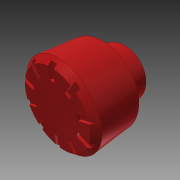
# Autodesk Inventor part: rotary_encoder_cnob
Saved by Autodesk Inventor 2014 (Build 180170000, 170)
## iProperties
Created: 2014-01-11
Part Number: rotary_encoder_cnob
Material: ABS Plastic
Document SubType Name: Modeling
Designer: buben
Density: 1.06 g/cm^3
Appearance: Light Red
Author: buben
Autodesk Inventor part; units mm, degrees
ref_plane "YZ Plane" through (0, 0, 0) normal (1, 0, 0) x (0, 1, 0)
ref_plane "XZ Plane" through (0, 0, 0) normal (0, 1, 0) x (-1, 0, 0)
ref_plane "XY Plane" through (0, 0, 0) normal (0, 0, 1) x (1, 0, 0)
sketch "Sketch1" plane through (0, 0, 0) normal (0, 1, 0) x (-1, 0, 0)
  circle A0 centre (0, 0) radius 7.5
  dimension "d0" = 15
  constraints: 1 centre point, 1 coincident
  measures "d0" diameter of A0
extrude "Extrusion1" add sketch "Sketch1" along normal blind 8
sketch "Sketch2" plane through (0, 8, 0) normal (0, 1, 0) x (1, 0, 0)
  circle A0 centre (0, 0) radius 7.5 projected
  circle A1 centre (0, 0) radius 5
  dimension "d3" = 10
  constraints: 1 centre point, 1 coincident
  measures "d3" diameter of A1
extrude "Extrusion2" add sketch "Sketch2" along normal blind 5 contours A1
sketch "Sketch3" plane through (0, 13, 0) normal (0, 1, 0) x (1, 0, 0)
  circle A0 centre (0, 0) radius 5 projected
  circle A1 centre (0, 0) radius 3 construction
  line L0 (-2.6295, 1.4442) -> (2.6295, 1.4442)
  arc A2 (-2.6295, 1.4442) -> (2.6295, 1.4442) centre (0, 0) ccw
  dimension "d6" = 6
  dimension "d7" = 5.259
  constraints: 4 point on circle, 2 centre point, 2 end point, 1 coincident, 1 concentric, 1 horizontal
  measures "d6" diameter of A1
  measures "d7" distance of L0.start L0.end
extrude "Extrusion3" cut sketch "Sketch3" against normal blind 11 contours L0 A2
chamfer "Chamfer1" distance 1 angle 45 1 edges at (7.5, 0, 0)
sketch "Sketch4" plane through (0, 0, 0) normal (0, -1, 0) x (1, 0, 0)
  circle A0 centre (0, 0) radius 6.5 construction
  line L0 (0, 0) -> (0, 6.5) construction
  line L1 (-0.5, 4.5) -> (0.5, 4.5)
  line L2 (0.5, 4.5) -> (0.5, 7.5)
  line L3 (0.5, 7.5) -> (-0.5, 7.5)
  line L4 (-0.5, 7.5) -> (-0.5, 4.5)
  circle A1 centre (0, 0) radius 7.5 construction
  line L5 (-3.0495, 3.3467) -> (-2.2405, 3.9345)
  line L6 (-2.2405, 3.9345) -> (-4.0039, 6.3615)
  line L7 (-4.0039, 6.3615) -> (-4.8129, 5.7737)
  line L8 (-4.8129, 5.7737) -> (-3.0495, 3.3467)
  line L9 (-4.4343, 0.915) -> (-4.1252, 1.8661)
  line L10 (-4.1252, 1.8661) -> (-6.9784, 2.7932)
  line L11 (-6.9784, 2.7932) -> (-7.2874, 1.8421)
  line L12 (-7.2874, 1.8421) -> (-4.4343, 0.915)
  line L13 (-4.1252, -1.8661) -> (-4.4343, -0.915)
  line L14 (-4.4343, -0.915) -> (-7.2874, -1.8421)
  line L15 (-7.2874, -1.8421) -> (-6.9784, -2.7932)
  line L16 (-6.9784, -2.7932) -> (-4.1252, -1.8661)
  line L17 (-2.2405, -3.9345) -> (-3.0495, -3.3467)
  line L18 (-3.0495, -3.3467) -> (-4.8129, -5.7737)
  line L19 (-4.8129, -5.7737) -> (-4.0039, -6.3615)
  line L20 (-4.0039, -6.3615) -> (-2.2405, -3.9345)
  line L21 (0.5, -4.5) -> (-0.5, -4.5)
  line L22 (-0.5, -4.5) -> (-0.5, -7.5)
  line L23 (-0.5, -7.5) -> (0.5, -7.5)
  line L24 (0.5, -7.5) -> (0.5, -4.5)
  line L25 (3.0495, -3.3467) -> (2.2405, -3.9345)
  line L26 (2.2405, -3.9345) -> (4.0039, -6.3615)
  line L27 (4.0039, -6.3615) -> (4.8129, -5.7737)
  line L28 (4.8129, -5.7737) -> (3.0495, -3.3467)
  line L29 (4.4343, -0.915) -> (4.1252, -1.8661)
  line L30 (4.1252, -1.8661) -> (6.9784, -2.7932)
  line L31 (6.9784, -2.7932) -> (7.2874, -1.8421)
  line L32 (7.2874, -1.8421) -> (4.4343, -0.915)
  line L33 (4.1252, 1.8661) -> (4.4343, 0.915)
  line L34 (4.4343, 0.915) -> (7.2874, 1.8421)
  line L35 (7.2874, 1.8421) -> (6.9784, 2.7932)
  line L36 (6.9784, 2.7932) -> (4.1252, 1.8661)
  line L37 (2.2405, 3.9345) -> (3.0495, 3.3467)
  line L38 (3.0495, 3.3467) -> (4.8129, 5.7737)
  line L39 (4.8129, 5.7737) -> (4.0039, 6.3615)
  line L40 (4.0039, 6.3615) -> (2.2405, 3.9345)
  point P0 (0, 4.5)
  point P1 (-2.645, 3.6406)
  point P2 (-4.2798, 1.3906)
  point P3 (-4.2798, -1.3906)
  point P4 (-2.645, -3.6406)
  point P5 (0, -4.5)
  point P6 (2.645, -3.6406)
  point P7 (4.2798, -1.3906)
  point P8 (4.2798, 1.3906)
  point P9 (2.645, 3.6406)
  dimension "d13" = 1
  dimension "d14" = 3
  dimension "d17" = 360
  constraints: 82 end point, 2 parallel, 1 horizontal, 1 midpoint, 1 perpendicular, 1 point on line, 1 tangent, 1 vertical, 1 vertical alignment, 92 other
  measures "d13" distance of L1.start L1.end
  measures "d14" distance of L1.end L2.end
extrude "Extrusion4" cut sketch "Sketch4" against normal blind 0.5
body "Solid1"
